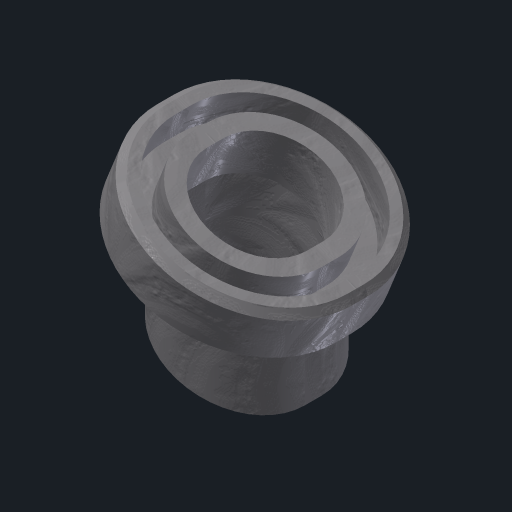
# Autodesk Inventor part: COMPUERTA_PLASTICO
Saved by Autodesk Inventor 2024.3 (Build 283343000, 343)
## iProperties
Created: 2024-07-04
Part Number: COMPUERTA_PLASTICO
Material: Steel, Mild, Welded
Document SubType Name: Modeling
Designer: Niler
Density: 7.85 g/cm^3
Appearance: Weld - Steel Mild
Author: Niler
Autodesk Inventor part; units mm, degrees
ref_plane "YZ Plane" through (0, 0, 0) normal (1, 0, 0) x (0, 1, 0)
ref_plane "XZ Plane" through (0, 0, 0) normal (0, 1, 0) x (-1, 0, 0)
ref_plane "XY Plane" through (0, 0, 0) normal (0, 0, 1) x (1, 0, 0)
sketch "Sketch1" plane through (0, 0, 0) normal (0, 1, 0) x (-1, 0, 0)
  line L0 (-101.5312, 175) -> (101.5312, 175)
  line L1 (101.5312, 175) -> (101.5312, -175)
  line L2 (101.5312, -175) -> (-101.5312, -175)
  line L3 (-101.5312, -175) -> (-101.5312, 175)
  line L4 (-101.5312, 175) -> (101.5312, -175) construction
  line L5 (101.5312, 175) -> (-101.5312, -175) construction
  point P0 (0, 0)
  dimension "d2" = 350
  constraints: 12 end point, 2 midpoint, 2 parallel, 1 horizontal, 1 perpendicular
  measures "d2" distance of L0.end L1.end
extrude "Extrusion1" add sketch "Sketch1" against normal blind 150
sketch "Sketch3" plane through (-101.5312, 0, 175) normal (0, 0, 1) x (-1, 0, 0)
  line L0 (0, 0) -> (-203.0624, 0) projected
  line L1 (-203.0624, 0) -> (-203.0624, 150) projected
  line L2 (-203.0624, 150) -> (0, 150) projected
  line L3 (0, 0) -> (0, 150) projected
  line L4 (0, 150) -> (-48.8156, 150)
  line L5 (0, 0) -> (47.3608, 0)
  line L6 (0, 0) -> (-203.0624, 81.2192)
  point P0 (-101.5312, 0)
  dimension "d7" = 158.2
  constraints: 6 end point, 2 horizontal, 1 point on line
  measures "d7" angle of L5 L6
extrude "Extrusion2" cut sketch "Sketch3" against normal through all contours L0 L1 L6
sketch "Sketch5" plane through (-101.5312, -150, 175) normal (0, 0, 1) x (1, 0, 0)
  line L0 (203.0624, 68.7808) -> (0, 150) projected
  line L1 (203.0624, 44.0093) -> (0, 125.2285)
  line L2 (0, 150) -> (0, 125.2285)
  line L3 (0, 150) -> (0, 0) projected
  line L4 (203.0624, 68.7808) -> (203.0624, 44.0093)
  line L5 (203.0624, 68.7808) -> (203.0624, 0) projected
  line L6 (203.0624, 0) -> (0, 0) projected
  point P0 (101.5312, 150)
  dimension "d13" = 23
  constraints: 8 end point, 1 parallel, 1 point on line, 1 vertical
  measures "d13" distance between parallel lines of L0 L1
extrude "Extrusion4" cut sketch "Sketch5" against normal through all contours L5 L6 L3 L1
sketch "Sketch4" plane through (0, 0, 0) normal (0, 1, 0) x (-1, 0, 0)
  line L0 (0, 2.5) -> (0, -2.5) construction
  line L1 (-20, 2.5) -> (-20, -2.5)
  line L2 (20, -2.5) -> (20, 2.5)
  arc A0 (20, 2.5) -> (-20, 2.5) centre (0, 2.5) ccw
  arc A1 (-20, -2.5) -> (20, -2.5) centre (0, -2.5) ccw
  line L3 (101.5312, -175) -> (-101.5312, -175) projected
  line L4 (101.5312, -175) -> (101.5312, 175) projected
  line L5 (-101.5312, 175) -> (101.5312, 175) projected
  line L6 (-101.5312, -175) -> (-101.5312, 175) projected
  line L7 (15, -2.5) -> (15, 2.5)
  arc A2 (15, 2.5) -> (-15, 2.5) centre (0, 2.5) ccw
  line L8 (-15, 2.5) -> (-15, -2.5)
  arc A3 (-15, -2.5) -> (15, -2.5) centre (0, -2.5) ccw
  point P0 (0, 0)
  dimension "d9" = 5
  dimension "d10" = 40
  dimension "d16" = 30
  constraints: 12 end point, 8 point on circle, 4 centre point, 4 tangent, 2 parallel, 1 midpoint, 1 vertical, 3 other
  measures "d9" distance of L0.start L0.end
  measures "d10" distance between parallel lines of L1 L2
  measures "d16" distance between parallel lines of L8 L7
extrude "Extrusion3" cut sketch "Sketch4" against normal through all
sketch "Sketch6" plane through (-20, -32.6101, 2.5) normal (0.3713678, 0.9284858, 0) x (0.9284858, -0.3713678, 0)
  line L0 (0, 5) -> (0, 0) projected
  ellipse E0 centre (21.5404, 0) end of major axis (43.0809, 0) minor radius 20 (0, 0) -> (43.0809, 0) ccw projected
  line L1 (43.0809, 0) -> (43.0809, 5) projected
  ellipse E1 centre (21.5404, 5) end of major axis (0, 5) minor radius 20 (43.0809, 5) -> (0, 5) ccw projected
  line L2 (37.6958, 5) -> (37.6958, 0) projected
  ellipse E2 centre (21.5404, 0) end of major axis (5.3851, 0) minor radius 15 (5.3851, 0) -> (37.6958, 0) ccw projected
  line L3 (5.3851, 0) -> (5.3851, 5) projected
  ellipse E3 centre (21.5404, 5) end of major axis (37.6958, 5) minor radius 15 (37.6958, 5) -> (5.3851, 5) ccw projected
  line L4 (-10, 0) -> (-10, 5)
  line L5 (53.0809, 5) -> (53.0809, 0)
  spline S0 degree 5 poles (-9.9999, 5) (-9.9999, 7.1264) (-9.8022, 9.2528) (-9.4067, 11.3546) (-7.4301, 18.2587) (-3.404, 24.3702) (0.2948, 27.9843) (8.9009, 33.5417) (18.9643, 35.4814) (24.1166, 35.4814) (34.18, 33.5417) (42.7861, 27.9843) (46.4849, 24.3702) (50.511, 18.2587) (52.4876, 11.3546) (52.8831, 9.2528) (53.0808, 7.1264) (53.0808, 5) knots 0 0 0 0 0 0 0.109959 0.109959 0.109959 0.369841 0.369841 0.369841 0.630159 0.630159 0.630159 0.890041 0.890041 0.890041 1 1 1 1 1 1
  spline S1 degree 5 poles (53.0808, 0) (53.0808, -2.1264) (52.8831, -4.2528) (52.4876, -6.3546) (50.511, -13.2587) (46.4849, -19.3702) (42.7861, -22.9843) (34.18, -28.5417) (24.1166, -30.4814) (18.9643, -30.4814) (8.9009, -28.5417) (0.2948, -22.9843) (-3.404, -19.3702) (-7.4301, -13.2587) (-9.4067, -6.3546) (-9.8022, -4.2528) (-9.9999, -2.1264) (-9.9999, 0) knots 0 0 0 0 0 0 0.109959 0.109959 0.109959 0.369841 0.369841 0.369841 0.630159 0.630159 0.630159 0.890041 0.890041 0.890041 1 1 1 1 1 1
  point P0 (6.4594, 2.5)
  dimension "d17" = 10
  constraints: 4 end point, 3 parallel, 2 horizontal alignment, 8 other
  measures "d17" distance between parallel lines of L0 L4
extrude "Extrusion5" add sketch "Sketch6" along normal blind 15 contours E1 L1 E0 L0 | L4 S0 L5 S1
sketch "Sketch7" plane through (-14.4295, -18.6829, 2.5) normal (0.3713678, 0.9284858, 0) x (0.9284858, -0.3713678, 0)
  line L0 (53.0809, 0) -> (53.0809, 5) projected
  spline S0 degree 5 poles (53.0809, 5) (53.0808, 7.1264) (52.8831, 9.2528) (52.4876, 11.3546) (50.511, 18.2587) (46.4849, 24.3702) (42.7861, 27.9843) (34.18, 33.5417) (24.1166, 35.4814) (18.9643, 35.4814) (8.9009, 33.5417) (0.2948, 27.9843) (-3.404, 24.3702) (-7.4301, 18.2587) (-9.4067, 11.3546) (-9.8022, 9.2528) (-9.9999, 7.1264) (-9.9999, 5) knots 0 0 0 0 0 0 0.109959 0.109959 0.109959 0.369841 0.369841 0.369841 0.630159 0.630159 0.630159 0.890041 0.890041 0.890041 1 1 1 1 1 1
  line L1 (-10, 5) -> (-10, 0) projected
  spline S1 degree 5 poles (-10, 0) (-9.9999, -2.1264) (-9.8022, -4.2528) (-9.4067, -6.3546) (-7.4301, -13.2587) (-3.404, -19.3702) (0.2948, -22.9843) (8.9009, -28.5417) (18.9643, -30.4814) (24.1166, -30.4814) (34.18, -28.5417) (42.7861, -22.9843) (46.4849, -19.3702) (50.511, -13.2587) (52.4876, -6.3546) (52.8831, -4.2528) (53.0808, -2.1264) (53.0809, 0) knots 0 0 0 0 0 0 0.109959 0.109959 0.109959 0.369841 0.369841 0.369841 0.630159 0.630159 0.630159 0.890041 0.890041 0.890041 1 1 1 1 1 1
  line L2 (5.3851, 0) -> (5.3851, 5) projected
  ellipse E0 centre (21.5404, 5) end of major axis (5.3851, 5) minor radius 15 (37.6958, 5) -> (5.3851, 5) ccw projected
  line L3 (37.6958, 5) -> (37.6958, 0) projected
  ellipse E1 centre (21.5404, 0) end of major axis (37.6958, 0) minor radius 15 (5.3851, 0) -> (37.6958, 0) ccw projected
  line L4 (48.0809, 0) -> (48.0809, 5)
  line L5 (-5, 5) -> (-5, 0)
  line L6 (42.6958, 0) -> (42.6958, 5)
  line L7 (0.3851, 5) -> (0.3851, 0)
  spline S2 degree 5 poles (48.0809, 4.9998) (48.0807, 9.0109) (47.2287, 13.0249) (45.5176, 16.7881) (40.65, 23.4461) (33.623, 27.7811) (29.7135, 29.2586) (21.5404, 30.7416) (13.3674, 29.2587) (9.4579, 27.7811) (2.431, 23.4461) (-2.4366, 16.7882) (-4.1476, 13.0251) (-4.9999, 9.0111) (-4.9999, 5) knots 0 0 0 0 0 0 0.247683 0.247683 0.247683 0.500001 0.500001 0.500001 0.75232 0.75232 0.75232 1 1 1 1 1 1
  spline S3 degree 5 poles (-5, 0.0002) (-4.9998, -4.0109) (-4.1478, -8.0249) (-2.4367, -11.7881) (2.4309, -18.4461) (9.4579, -22.7811) (13.3674, -24.2586) (21.5404, -25.7416) (29.7135, -24.2586) (33.623, -22.7811) (40.65, -18.4461) (45.5176, -11.7881) (47.2287, -8.0249) (48.0807, -4.0109) (48.0809, 0.0002) knots 0 0 0 0 0 0 0.247682 0.247682 0.247682 0.5 0.5 0.5 0.752318 0.752318 0.752318 1 1 1 1 1 1
  spline S4 degree 5 poles (42.6957, 5) (42.6957, 6.4099) (42.5645, 7.8197) (42.3021, 9.2132) (40.9833, 13.8173) (38.2917, 17.8905) (35.8139, 20.3012) (30.0335, 24.0241) (23.2767, 25.3241) (19.8042, 25.3241) (13.0474, 24.0241) (7.267, 20.3012) (4.7892, 17.8905) (2.0976, 13.8173) (0.7788, 9.2132) (0.5164, 7.8197) (0.3852, 6.4099) (0.3852, 5) knots 0 0 0 0 0 0 0.109014 0.109014 0.109014 0.368803 0.368803 0.368803 0.631197 0.631197 0.631197 0.890986 0.890986 0.890986 1 1 1 1 1 1
  spline S5 degree 5 poles (0.3852, 0) (0.3852, -1.4099) (0.5164, -2.8197) (0.7788, -4.2132) (2.0976, -8.8173) (4.7892, -12.8905) (7.267, -15.3012) (13.0474, -19.0241) (19.8042, -20.3241) (23.2767, -20.3241) (30.0335, -19.0241) (35.8139, -15.3012) (38.2917, -12.8905) (40.9833, -8.8173) (42.3021, -4.2132) (42.5645, -2.8197) (42.6957, -1.4099) (42.6957, 0) knots 0 0 0 0 0 0 0.109014 0.109014 0.109014 0.368803 0.368803 0.368803 0.631197 0.631197 0.631197 0.890986 0.890986 0.890986 1 1 1 1 1 1
  point P0 (6.4594, 2.5)
  dimension "d20" = 5
  dimension "d21" = 5
  constraints: 8 end point, 6 horizontal alignment, 6 parallel, 10 other
extrude "Extrusion6" cut sketch "Sketch7" against normal blind 10 contours S3 L5 S2 L4
chamfer "Chamfer1" distance 2 angle 45 4 edges at (5.5705, -26.6823, 32.5001) (34.8554, -38.3954, 0) (5.5705, -26.6823, -32.5001) (-23.7143, -14.9692, 0)
body "Solid1"
